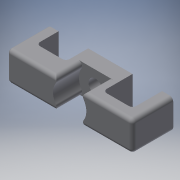
# Autodesk Inventor part: WireClampDual
Saved by Autodesk Inventor 2017 (Build 210142000, 142)
## iProperties
Created: 2015-07-07
Part Number: WireClampDual
Material: Generic
Document SubType Name: Modeling
Designer: Dale
Density: 1 g/cm^3
Appearance: Default
Author: Dale
Autodesk Inventor part; units mm, degrees
ref_plane "YZ Plane" through (0, 0, 0) normal (1, 0, 0) x (0, 1, 0)
ref_plane "XZ Plane" through (0, 0, 0) normal (0, 1, 0) x (-1, 0, 0)
ref_plane "XY Plane" through (0, 0, 0) normal (0, 0, 1) x (1, 0, 0)
sketch "Sketch1" plane through (0, 0, 0) normal (0, 0, 1) x (1, 0, 0)
  line L0 (0, 4) -> (16, 4)
  line L1 (17, 3) -> (17, -3)
  line L2 (16, -4) -> (0, -4)
  arc A0 (17, 3) -> (16, 4) centre (16, 3) ccw
  arc A1 (16, -4) -> (17, -3) centre (16, -3) ccw
  line L3 (0, 4) -> (-16, 4)
  line L4 (-17, 3) -> (-17, -3)
  line L5 (-16, -4) -> (0, -4)
  arc A2 (-16, 4) -> (-17, 3) centre (-16, 3) ccw
  arc A3 (-17, -3) -> (-16, -4) centre (-16, -3) ccw
  line L6 (0, 4) -> (0, -4)
  point P0 (0, 0)
  point P1 (0, 0)
  dimension "d1" = 17
  dimension "d2" = 1
  dimension "d17" = 17
  dimension "d18" = 4
  dimension "d19" = 4
  dimension "d20" = 1
  dimension "d21" = 8
  dimension "d22" = 4
  constraints: 14 end point, 8 point on circle, 8 tangent, 4 centre point, 3 coincident, 3 horizontal, 2 equal radius, 1 parallel, 1 perpendicular, 1 vertical
  measures "d1" distance from line of point (0, 0) L1
  measures "d2" radius of A0
  measures "d17" distance from line of point (0, 0) L4
  measures "d18" distance of L0.start point (0, 0)
  measures "d19" distance of L2.end point (0, 0)
  measures "d20" radius of A2
  measures "d21" distance between parallel lines of L0 L2
  measures "d22" distance from line of point (0, 0) L0
extrude "Extrusion1" add sketch "Sketch1" along normal blind 11
sketch "Sketch5" plane through (-16, -4, 0) normal (0, -1, 0) x (1, 0, 0)
  line L0 (0, 0) -> (32, 0) projected
  line L1 (22, 0) -> (30, 0)
  line L2 (30, 0) -> (30, 7)
  line L3 (29, 8) -> (23, 8)
  line L4 (22, 7) -> (22, 0)
  line L5 (33, 0) -> (33, 11) projected
  arc A0 (23, 8) -> (22, 7) centre (23, 7) ccw
  arc A1 (30, 7) -> (29, 8) centre (29, 7) ccw
  line L6 (3, 6) -> (9, 6)
  line L7 (10, 5) -> (10, 0)
  line L8 (10, 0) -> (2, 0)
  line L9 (2, 0) -> (2, 5)
  line L10 (-1, 0) -> (-1, 11) projected
  line L11 (32, 0) -> (0, 0) projected
  arc A2 (3, 6) -> (2, 5) centre (3, 5) ccw
  arc A3 (10, 5) -> (9, 6) centre (9, 5) ccw
  point P0 (16, 0)
  point P1 (10, 6)
  dimension "d28" = 3
  dimension "d29" = 8
  dimension "d30" = 8
  dimension "d31" = 1
  dimension "d34" = 3
  dimension "d35" = 8
  dimension "d36" = 6
  dimension "d37" = 1
  constraints: 16 end point, 8 point on circle, 8 tangent, 4 centre point, 4 parallel, 3 point on line, 2 equal radius, 2 horizontal, 2 perpendicular, 1 collinear
  measures "d28" distance between parallel lines of L5 L2
  measures "d29" distance between parallel lines of L0 L3
  measures "d30" distance between parallel lines of L4 L2
  measures "d31" radius of A0
  measures "d34" distance between parallel lines of L10 L9
  measures "d35" distance between parallel lines of L7 L9
  measures "d36" distance of point (10, 6) L7.end
  measures "d37" radius of A2
extrude "Extrusion5" cut sketch "Sketch5" against normal through all
sketch "Sketch3" plane through (-16, -3, 11) normal (0, 0, 1) x (1, 0, 0)
  circle A0 centre (16, 3) radius 4.5
  dimension "d38" = 9
  constraints: 1 centre point, 1 coincident
  measures "d38" diameter of A0
extrude "Extrusion3" cut sketch "Sketch3" against normal blind 7
sketch "Sketch4" plane through (-16, -3, 4) normal (0, 0, 1) x (1, 0, 0)
  circle A0 centre (16, 3) radius 1.905
  dimension "d13" = 3.81
  constraints: 1 centre point, 1 coincident
  measures "d13" diameter of A0
extrude "Extrusion4" cut sketch "Sketch4" against normal through all
fillet "Fillet2" radius 1 10 edges at (9.0308, -4, 11) (-16.7071, -3.7071, 11) (-17, 0, 11) (-16.7071, 3.7071, 11) (-9.0308, 4, 11) (16.7071, -3.7071, 11) (17, 0, 11) (16.7071, 3.7071, 11) (2.0616, -4, 7.5) (-2.0616, 4, 7.5)
body "Solid1"
